Autodesk Fusion 360 part; units mm, degrees
note: some values were not read from the file. Chosen so that the rebuilt part matches the saved one: which pieces of a blend or face edit are solid.
(part 3 of 4)
  arc A691 (-206.3206, 126.4632) -> (-207.0079, 125.7759) centre (-206.5811, 126.0364) ccw
  arc A692 (-206.3206, 126.4632) -> (-206.1643, 126.4193) centre (-206.1643, 126.7193) ccw
  line L408 (-206.1643, 126.4193) -> (-205.2639, 126.4193)
  line L409 (-205.2639, 126.4193) -> (-204.3636, 126.4193)
  arc A693 (-204.3636, 126.4193) -> (-204.2073, 126.4632) centre (-204.3636, 126.7193) ccw
  arc A694 (-203.52, 125.7759) -> (-204.2073, 126.4632) centre (-203.9468, 126.0364) ccw
  arc A695 (-203.52, 125.7759) -> (-203.5639, 125.6196) centre (-203.2639, 125.6196) ccw
  line L410 (-203.5639, 125.6196) -> (-203.5639, 124.9193)
  line L411 (-203.5639, 124.9193) -> (-203.5639, 124.2189)
  arc A696 (-203.5639, 124.2189) -> (-203.52, 124.0626) centre (-203.2639, 124.2189) ccw
  arc A697 (-223.2573, 123.3754) -> (-222.57, 124.0626) centre (-222.9968, 123.8021) ccw
  arc A698 (-223.2573, 123.3754) -> (-223.4136, 123.4193) centre (-223.4135, 123.1196) ccw
  line L412 (-223.4136, 123.4193) -> (-224.3139, 123.4193)
  line L413 (-224.3139, 123.4193) -> (-225.2143, 123.4193)
  arc A699 (-225.2143, 123.4193) -> (-225.3706, 123.3754) centre (-225.2143, 123.1193) ccw
  arc A700 (-226.0579, 124.0626) -> (-225.3706, 123.3754) centre (-225.6311, 123.8021) ccw
  arc A701 (-226.0579, 124.0626) -> (-226.0139, 124.2189) centre (-226.3139, 124.2189) ccw
  line L414 (-226.0139, 124.2189) -> (-226.0139, 124.9193)
  line L415 (-226.0139, 124.9193) -> (-226.0139, 125.6196)
  arc A702 (-226.0139, 125.6196) -> (-226.0579, 125.7759) centre (-226.3139, 125.6196) ccw
  arc A703 (-225.3706, 126.4632) -> (-226.0579, 125.7759) centre (-225.6311, 126.0364) ccw
  arc A704 (-225.3706, 126.4632) -> (-225.2143, 126.4193) centre (-225.2143, 126.7193) ccw
  line L416 (-225.2143, 126.4193) -> (-224.3139, 126.4193)
  line L417 (-224.3139, 126.4193) -> (-223.4136, 126.4193)
  arc A705 (-223.4136, 126.4193) -> (-223.2573, 126.4632) centre (-223.4136, 126.7193) ccw
  arc A706 (-222.57, 125.7759) -> (-223.2573, 126.4632) centre (-222.9968, 126.0364) ccw
  arc A707 (-222.57, 125.7759) -> (-222.6139, 125.6196) centre (-222.3139, 125.6196) ccw
  line L418 (-222.6139, 125.6196) -> (-222.6139, 124.9193)
  line L419 (-222.6139, 124.9193) -> (-222.6139, 124.2189)
  arc A708 (-222.6139, 124.2189) -> (-222.57, 124.0626) centre (-222.3139, 124.2189) ccw
  circle A709 centre (-191.2939, 119.8393) radius 0.875
  circle A710 centre (-200.1839, 119.8393) radius 0.875
  circle A711 centre (-205.2639, 119.8393) radius 1.9939
  circle A712 centre (-201.4539, 117.2993) radius 1.5
  circle A713 centre (-188.7539, 114.7593) radius 1.5
  circle A714 centre (-210.3439, 119.8393) radius 0.875
  circle A715 centre (-219.2339, 119.8393) radius 0.875
  circle A716 centre (-224.3139, 119.8393) radius 1.9939
  circle A717 centre (-220.5039, 117.2993) radius 1.5
  circle A718 centre (-207.8039, 114.7593) radius 1.5
  arc A719 (-156.5823, 104.3254) -> (-155.895, 105.0126) centre (-156.3218, 104.7521) ccw
  arc A720 (-156.5823, 104.3254) -> (-156.7386, 104.3693) centre (-156.7385, 104.0696) ccw
  line L420 (-156.7386, 104.3693) -> (-157.6389, 104.3693)
  line L421 (-157.6389, 104.3693) -> (-158.5393, 104.3693)
  arc A721 (-158.5393, 104.3693) -> (-158.6956, 104.3254) centre (-158.5393, 104.0693) ccw
  arc A722 (-159.3829, 105.0126) -> (-158.6956, 104.3254) centre (-158.9561, 104.7521) ccw
  arc A723 (-159.3829, 105.0126) -> (-159.3389, 105.1689) centre (-159.6389, 105.1689) ccw
  line L422 (-159.3389, 105.1689) -> (-159.3389, 105.8693)
  line L423 (-159.3389, 105.8693) -> (-159.3389, 106.5696)
  arc A724 (-159.3389, 106.5696) -> (-159.3829, 106.7259) centre (-159.6389, 106.5696) ccw
  arc A725 (-158.6956, 107.4132) -> (-159.3829, 106.7259) centre (-158.9561, 106.9864) ccw
  arc A726 (-158.6956, 107.4132) -> (-158.5393, 107.3693) centre (-158.5393, 107.6693) ccw
  line L424 (-158.5393, 107.3693) -> (-157.6389, 107.3693)
  line L425 (-157.6389, 107.3693) -> (-156.7386, 107.3693)
  arc A727 (-156.7386, 107.3693) -> (-156.5823, 107.4132) centre (-156.7386, 107.6693) ccw
  arc A728 (-155.895, 106.7259) -> (-156.5823, 107.4132) centre (-156.3218, 106.9864) ccw
  arc A729 (-155.895, 106.7259) -> (-155.9389, 106.5696) centre (-155.6389, 106.5696) ccw
  line L426 (-155.9389, 106.5696) -> (-155.9389, 105.8693)
  line L427 (-155.9389, 105.8693) -> (-155.9389, 105.1689)
  arc A730 (-155.9389, 105.1689) -> (-155.895, 105.0126) centre (-155.6389, 105.1689) ccw
  arc A731 (-175.6323, 104.3254) -> (-174.945, 105.0126) centre (-175.3718, 104.7521) ccw
  arc A732 (-175.6323, 104.3254) -> (-175.7886, 104.3693) centre (-175.7885, 104.0696) ccw
  line L428 (-175.7886, 104.3693) -> (-176.6889, 104.3693)
  line L429 (-176.6889, 104.3693) -> (-177.5893, 104.3693)
  arc A733 (-177.5893, 104.3693) -> (-177.7456, 104.3254) centre (-177.5893, 104.0693) ccw
  arc A734 (-178.4329, 105.0126) -> (-177.7456, 104.3254) centre (-178.0061, 104.7521) ccw
  arc A735 (-178.4329, 105.0126) -> (-178.3889, 105.1689) centre (-178.6889, 105.1689) ccw
  line L430 (-178.3889, 105.1689) -> (-178.3889, 105.8693)
  line L431 (-178.3889, 105.8693) -> (-178.3889, 106.5696)
  arc A736 (-178.3889, 106.5696) -> (-178.4329, 106.7259) centre (-178.6889, 106.5696) ccw
  arc A737 (-177.7456, 107.4132) -> (-178.4329, 106.7259) centre (-178.0061, 106.9864) ccw
  arc A738 (-177.7456, 107.4132) -> (-177.5893, 107.3693) centre (-177.5893, 107.6693) ccw
  line L432 (-177.5893, 107.3693) -> (-176.6889, 107.3693)
  line L433 (-176.6889, 107.3693) -> (-175.7886, 107.3693)
  arc A739 (-175.7886, 107.3693) -> (-175.6323, 107.4132) centre (-175.7886, 107.6693) ccw
  arc A740 (-174.945, 106.7259) -> (-175.6323, 107.4132) centre (-175.3718, 106.9864) ccw
  arc A741 (-174.945, 106.7259) -> (-174.9889, 106.5696) centre (-174.6889, 106.5696) ccw
  line L434 (-174.9889, 106.5696) -> (-174.9889, 105.8693)
  line L435 (-174.9889, 105.8693) -> (-174.9889, 105.1689)
  arc A742 (-174.9889, 105.1689) -> (-174.945, 105.0126) centre (-174.6889, 105.1689) ccw
  circle A743 centre (-152.5589, 100.7893) radius 0.875
  circle A744 centre (-153.8289, 98.2493) radius 1.5
  circle A745 centre (-157.6389, 100.7893) radius 1.9939
  circle A746 centre (-162.7189, 100.7893) radius 0.875
  circle A747 centre (-171.6089, 100.7893) radius 0.875
  circle A748 centre (-172.8789, 98.2493) radius 1.5
  circle A749 centre (-176.6889, 100.7893) radius 1.9939
  circle A750 centre (-181.7689, 100.7893) radius 0.875
  arc A751 (-194.6823, 104.3254) -> (-193.995, 105.0126) centre (-194.4218, 104.7521) ccw
  arc A752 (-194.6823, 104.3254) -> (-194.8386, 104.3693) centre (-194.8385, 104.0696) ccw
  line L436 (-194.8386, 104.3693) -> (-195.7389, 104.3693)
  line L437 (-195.7389, 104.3693) -> (-196.6393, 104.3693)
  arc A753 (-196.6393, 104.3693) -> (-196.7956, 104.3254) centre (-196.6393, 104.0693) ccw
  arc A754 (-197.4829, 105.0126) -> (-196.7956, 104.3254) centre (-197.0561, 104.7521) ccw
  arc A755 (-197.4829, 105.0126) -> (-197.4389, 105.1689) centre (-197.7389, 105.1689) ccw
  line L438 (-197.4389, 105.1689) -> (-197.4389, 105.8693)
  line L439 (-197.4389, 105.8693) -> (-197.4389, 106.5696)
  arc A756 (-197.4389, 106.5696) -> (-197.4829, 106.7259) centre (-197.7389, 106.5696) ccw
  arc A757 (-196.7956, 107.4132) -> (-197.4829, 106.7259) centre (-197.0561, 106.9864) ccw
  arc A758 (-196.7956, 107.4132) -> (-196.6393, 107.3693) centre (-196.6393, 107.6693) ccw
  line L440 (-196.6393, 107.3693) -> (-195.7389, 107.3693)
  line L441 (-195.7389, 107.3693) -> (-194.8386, 107.3693)
  arc A759 (-194.8386, 107.3693) -> (-194.6823, 107.4132) centre (-194.8386, 107.6693) ccw
  arc A760 (-193.995, 106.7259) -> (-194.6823, 107.4132) centre (-194.4218, 106.9864) ccw
  arc A761 (-193.995, 106.7259) -> (-194.0389, 106.5696) centre (-193.7389, 106.5696) ccw
  line L442 (-194.0389, 106.5696) -> (-194.0389, 105.8693)
  line L443 (-194.0389, 105.8693) -> (-194.0389, 105.1689)
  arc A762 (-194.0389, 105.1689) -> (-193.995, 105.0126) centre (-193.7389, 105.1689) ccw
  arc A763 (-213.7323, 104.3254) -> (-213.045, 105.0126) centre (-213.4718, 104.7521) ccw
  arc A764 (-213.7323, 104.3254) -> (-213.8886, 104.3693) centre (-213.8885, 104.0696) ccw
  line L444 (-213.8886, 104.3693) -> (-214.7889, 104.3693)
  line L445 (-214.7889, 104.3693) -> (-215.6893, 104.3693)
  arc A765 (-215.6893, 104.3693) -> (-215.8456, 104.3254) centre (-215.6893, 104.0693) ccw
  arc A766 (-216.5329, 105.0126) -> (-215.8456, 104.3254) centre (-216.1061, 104.7521) ccw
  arc A767 (-216.5329, 105.0126) -> (-216.4889, 105.1689) centre (-216.7889, 105.1689) ccw
  line L446 (-216.4889, 105.1689) -> (-216.4889, 105.8693)
  line L447 (-216.4889, 105.8693) -> (-216.4889, 106.5696)
  arc A768 (-216.4889, 106.5696) -> (-216.5329, 106.7259) centre (-216.7889, 106.5696) ccw
  arc A769 (-215.8456, 107.4132) -> (-216.5329, 106.7259) centre (-216.1061, 106.9864) ccw
  arc A770 (-215.8456, 107.4132) -> (-215.6893, 107.3693) centre (-215.6893, 107.6693) ccw
  line L448 (-215.6893, 107.3693) -> (-214.7889, 107.3693)
  line L449 (-214.7889, 107.3693) -> (-213.8886, 107.3693)
  arc A771 (-213.8886, 107.3693) -> (-213.7323, 107.4132) centre (-213.8886, 107.6693) ccw
  arc A772 (-213.045, 106.7259) -> (-213.7323, 107.4132) centre (-213.4718, 106.9864) ccw
  arc A773 (-213.045, 106.7259) -> (-213.0889, 106.5696) centre (-212.7889, 106.5696) ccw
  line L450 (-213.0889, 106.5696) -> (-213.0889, 105.8693)
  line L451 (-213.0889, 105.8693) -> (-213.0889, 105.1689)
  arc A774 (-213.0889, 105.1689) -> (-213.045, 105.0126) centre (-212.7889, 105.1689) ccw
  circle A775 centre (-190.6589, 100.7893) radius 0.875
  circle A776 centre (-195.7389, 100.7893) radius 1.9939
  circle A777 centre (-191.9289, 98.2493) radius 1.5
  circle A778 centre (-200.8189, 100.7893) radius 0.875
  circle A779 centre (-209.7089, 100.7893) radius 0.875
  circle A780 centre (-214.7889, 100.7893) radius 1.9939
  circle A781 centre (-210.9789, 98.2493) radius 1.5
  circle A782 centre (-219.8689, 100.7893) radius 0.875
  arc A783 (-242.3073, 123.3754) -> (-241.62, 124.0626) centre (-242.0468, 123.8021) ccw
  arc A784 (-242.3073, 123.3754) -> (-242.4636, 123.4193) centre (-242.4635, 123.1196) ccw
  line L452 (-242.4636, 123.4193) -> (-243.3639, 123.4193)
  line L453 (-243.3639, 123.4193) -> (-244.2643, 123.4193)
  arc A785 (-244.2643, 123.4193) -> (-244.4206, 123.3754) centre (-244.2643, 123.1193) ccw
  arc A786 (-245.1079, 124.0626) -> (-244.4206, 123.3754) centre (-244.6811, 123.8021) ccw
  arc A787 (-245.1079, 124.0626) -> (-245.0639, 124.2189) centre (-245.3639, 124.2189) ccw
  line L454 (-245.0639, 124.2189) -> (-245.0639, 124.9193)
  line L455 (-245.0639, 124.9193) -> (-245.0639, 125.6196)
  arc A788 (-245.0639, 125.6196) -> (-245.1079, 125.7759) centre (-245.3639, 125.6196) ccw
  arc A789 (-244.4206, 126.4632) -> (-245.1079, 125.7759) centre (-244.6811, 126.0364) ccw
  arc A790 (-244.4206, 126.4632) -> (-244.2643, 126.4193) centre (-244.2643, 126.7193) ccw
  line L456 (-244.2643, 126.4193) -> (-243.3639, 126.4193)
  line L457 (-243.3639, 126.4193) -> (-242.4636, 126.4193)
  arc A791 (-242.4636, 126.4193) -> (-242.3073, 126.4632) centre (-242.4636, 126.7193) ccw
  arc A792 (-241.62, 125.7759) -> (-242.3073, 126.4632) centre (-242.0468, 126.0364) ccw
  arc A793 (-241.62, 125.7759) -> (-241.6639, 125.6196) centre (-241.3639, 125.6196) ccw
  line L458 (-241.6639, 125.6196) -> (-241.6639, 124.9193)
  line L459 (-241.6639, 124.9193) -> (-241.6639, 124.2189)
  arc A794 (-241.6639, 124.2189) -> (-241.62, 124.0626) centre (-241.3639, 124.2189) ccw
  arc A795 (-261.3573, 123.3754) -> (-260.67, 124.0626) centre (-261.0968, 123.8021) ccw
  arc A796 (-261.3573, 123.3754) -> (-261.5136, 123.4193) centre (-261.5135, 123.1196) ccw
  line L460 (-261.5136, 123.4193) -> (-262.4139, 123.4193)
  line L461 (-262.4139, 123.4193) -> (-263.3143, 123.4193)
  arc A797 (-263.3143, 123.4193) -> (-263.4706, 123.3754) centre (-263.3143, 123.1193) ccw
  arc A798 (-264.1579, 124.0626) -> (-263.4706, 123.3754) centre (-263.7311, 123.8021) ccw
  arc A799 (-264.1579, 124.0626) -> (-264.1139, 124.2189) centre (-264.4139, 124.2189) ccw
  line L462 (-264.1139, 124.2189) -> (-264.1139, 124.9193)
  line L463 (-264.1139, 124.9193) -> (-264.1139, 125.6196)
  arc A800 (-264.1139, 125.6196) -> (-264.1579, 125.7759) centre (-264.4139, 125.6196) ccw
  arc A801 (-263.4706, 126.4632) -> (-264.1579, 125.7759) centre (-263.7311, 126.0364) ccw
  arc A802 (-263.4706, 126.4632) -> (-263.3143, 126.4193) centre (-263.3143, 126.7193) ccw
  line L464 (-263.3143, 126.4193) -> (-262.4139, 126.4193)
  line L465 (-262.4139, 126.4193) -> (-261.5136, 126.4193)
  arc A803 (-261.5136, 126.4193) -> (-261.3573, 126.4632) centre (-261.5136, 126.7193) ccw
  arc A804 (-260.67, 125.7759) -> (-261.3573, 126.4632) centre (-261.0968, 126.0364) ccw
  arc A805 (-260.67, 125.7759) -> (-260.7139, 125.6196) centre (-260.4139, 125.6196) ccw
  line L466 (-260.7139, 125.6196) -> (-260.7139, 124.9193)
  line L467 (-260.7139, 124.9193) -> (-260.7139, 124.2189)
  arc A806 (-260.7139, 124.2189) -> (-260.67, 124.0626) centre (-260.4139, 124.2189) ccw
  circle A807 centre (-229.3939, 119.8393) radius 0.875
  circle A808 centre (-238.2839, 119.8393) radius 0.875
  circle A809 centre (-243.3639, 119.8393) radius 1.9939
  circle A810 centre (-239.5539, 117.2993) radius 1.5
  circle A811 centre (-226.8539, 114.7593) radius 1.5
  circle A812 centre (-245.9039, 114.7593) radius 1.5
  circle A813 centre (-248.4439, 119.8393) radius 0.875
  circle A814 centre (-257.3339, 119.8393) radius 0.875
  circle A815 centre (-262.4139, 119.8393) radius 1.9939
  circle A816 centre (-258.6039, 117.2993) radius 1.5
  circle A817 centre (-264.9539, 114.7593) radius 1.5
  arc A818 (-283.2079, 124.0626) -> (-282.5206, 123.3754) centre (-282.7811, 123.8021) ccw
  arc A819 (-283.2079, 124.0626) -> (-283.1639, 124.2189) centre (-283.4639, 124.2189) ccw
  line L468 (-283.1639, 124.2189) -> (-283.1639, 124.9193)
  line L469 (-283.1639, 124.9193) -> (-283.1639, 125.6196)
  arc A820 (-283.1639, 125.6196) -> (-283.2079, 125.7759) centre (-283.4639, 125.6196) ccw
  arc A821 (-282.5206, 126.4632) -> (-283.2079, 125.7759) centre (-282.7811, 126.0364) ccw
  arc A822 (-282.5206, 126.4632) -> (-282.3643, 126.4193) centre (-282.3643, 126.7193) ccw
  line L470 (-282.3643, 126.4193) -> (-281.4639, 126.4193)
  line L471 (-281.4639, 126.4193) -> (-280.5636, 126.4193)
  arc A823 (-280.5636, 126.4193) -> (-280.4073, 126.4632) centre (-280.5636, 126.7193) ccw
  arc A824 (-279.72, 125.7759) -> (-280.4073, 126.4632) centre (-280.1468, 126.0364) ccw
  arc A825 (-279.72, 125.7759) -> (-279.7639, 125.6196) centre (-279.4639, 125.6196) ccw
  line L472 (-279.7639, 125.6196) -> (-279.7639, 124.9193)
  line L473 (-279.7639, 124.9193) -> (-279.7639, 124.2189)
  arc A826 (-279.7639, 124.2189) -> (-279.72, 124.0626) centre (-279.4639, 124.2189) ccw
  arc A827 (-280.4073, 123.3754) -> (-279.72, 124.0626) centre (-280.1468, 123.8021) ccw
  arc A828 (-280.4073, 123.3754) -> (-280.5636, 123.4193) centre (-280.5635, 123.1196) ccw
  line L474 (-280.5636, 123.4193) -> (-281.4639, 123.4193)
  line L475 (-281.4639, 123.4193) -> (-282.3643, 123.4193)
  arc A829 (-282.3643, 123.4193) -> (-282.5206, 123.3754) centre (-282.3643, 123.1193) ccw
  arc A830 (-302.2579, 124.0626) -> (-301.5706, 123.3754) centre (-301.8311, 123.8021) ccw
  arc A831 (-302.2579, 124.0626) -> (-302.2139, 124.2189) centre (-302.5139, 124.2189) ccw
  line L476 (-302.2139, 124.2189) -> (-302.2139, 124.9193)
  line L477 (-302.2139, 124.9193) -> (-302.2139, 125.6196)
  arc A832 (-302.2139, 125.6196) -> (-302.2579, 125.7759) centre (-302.5139, 125.6196) ccw
  arc A833 (-301.5706, 126.4632) -> (-302.2579, 125.7759) centre (-301.8311, 126.0364) ccw
  arc A834 (-301.5706, 126.4632) -> (-301.4143, 126.4193) centre (-301.4143, 126.7193) ccw
  line L478 (-301.4143, 126.4193) -> (-300.5139, 126.4193)
  line L479 (-300.5139, 126.4193) -> (-299.6136, 126.4193)
  arc A835 (-299.6136, 126.4193) -> (-299.4573, 126.4632) centre (-299.6136, 126.7193) ccw
  arc A836 (-298.77, 125.7759) -> (-299.4573, 126.4632) centre (-299.1968, 126.0364) ccw
  arc A837 (-298.77, 125.7759) -> (-298.8139, 125.6196) centre (-298.5139, 125.6196) ccw
  line L480 (-298.8139, 125.6196) -> (-298.8139, 124.9193)
  line L481 (-298.8139, 124.9193) -> (-298.8139, 124.2189)
  arc A838 (-298.8139, 124.2189) -> (-298.77, 124.0626) centre (-298.5139, 124.2189) ccw
  arc A839 (-299.4573, 123.3754) -> (-298.77, 124.0626) centre (-299.1968, 123.8021) ccw
  arc A840 (-299.4573, 123.3754) -> (-299.6136, 123.4193) centre (-299.6135, 123.1196) ccw
  line L482 (-299.6136, 123.4193) -> (-300.5139, 123.4193)
  line L483 (-300.5139, 123.4193) -> (-301.4143, 123.4193)
  arc A841 (-301.4143, 123.4193) -> (-301.5706, 123.3754) centre (-301.4143, 123.1193) ccw
  circle A842 centre (-267.4939, 119.8393) radius 0.875
  circle A843 centre (-276.3839, 119.8393) radius 0.875
  circle A844 centre (-281.4639, 119.8393) radius 1.9939
  circle A845 centre (-277.6539, 117.2993) radius 1.5
  circle A846 centre (-284.0039, 114.7593) radius 1.5
  circle A847 centre (-286.5439, 119.8393) radius 0.875
  circle A848 centre (-295.4339, 119.8393) radius 0.875
  circle A849 centre (-300.5139, 119.8393) radius 1.9939
  circle A850 centre (-296.7039, 117.2993) radius 1.5
  circle A851 centre (-303.0539, 114.7593) radius 1.5
  arc A852 (-232.7823, 104.3254) -> (-232.095, 105.0126) centre (-232.5218, 104.7521) ccw
  arc A853 (-232.7823, 104.3254) -> (-232.9386, 104.3693) centre (-232.9385, 104.0696) ccw
  line L484 (-232.9386, 104.3693) -> (-233.8389, 104.3693)
  line L485 (-233.8389, 104.3693) -> (-234.7393, 104.3693)
  arc A854 (-234.7393, 104.3693) -> (-234.8956, 104.3254) centre (-234.7393, 104.0693) ccw
  arc A855 (-235.5829, 105.0126) -> (-234.8956, 104.3254) centre (-235.1561, 104.7521) ccw
  arc A856 (-235.5829, 105.0126) -> (-235.5389, 105.1689) centre (-235.8389, 105.1689) ccw
  line L486 (-235.5389, 105.1689) -> (-235.5389, 105.8693)
  line L487 (-235.5389, 105.8693) -> (-235.5389, 106.5696)
  arc A857 (-235.5389, 106.5696) -> (-235.5829, 106.7259) centre (-235.8389, 106.5696) ccw
  arc A858 (-234.8956, 107.4132) -> (-235.5829, 106.7259) centre (-235.1561, 106.9864) ccw
  arc A859 (-234.8956, 107.4132) -> (-234.7393, 107.3693) centre (-234.7393, 107.6693) ccw
  line L488 (-234.7393, 107.3693) -> (-233.8389, 107.3693)
  line L489 (-233.8389, 107.3693) -> (-232.9386, 107.3693)
  arc A860 (-232.9386, 107.3693) -> (-232.7823, 107.4132) centre (-232.9386, 107.6693) ccw
  arc A861 (-232.095, 106.7259) -> (-232.7823, 107.4132) centre (-232.5218, 106.9864) ccw
  arc A862 (-232.095, 106.7259) -> (-232.1389, 106.5696) centre (-231.8389, 106.5696) ccw
  line L490 (-232.1389, 106.5696) -> (-232.1389, 105.8693)
  line L491 (-232.1389, 105.8693) -> (-232.1389, 105.1689)
  arc A863 (-232.1389, 105.1689) -> (-232.095, 105.0126) centre (-231.8389, 105.1689) ccw
  arc A864 (-251.8323, 104.3254) -> (-251.145, 105.0126) centre (-251.5718, 104.7521) ccw
  arc A865 (-251.8323, 104.3254) -> (-251.9886, 104.3693) centre (-251.9885, 104.0696) ccw
  line L492 (-251.9886, 104.3693) -> (-252.8889, 104.3693)
  line L493 (-252.8889, 104.3693) -> (-253.7893, 104.3693)
  arc A866 (-253.7893, 104.3693) -> (-253.9456, 104.3254) centre (-253.7893, 104.0693) ccw
  arc A867 (-254.6329, 105.0126) -> (-253.9456, 104.3254) centre (-254.2061, 104.7521) ccw
  arc A868 (-254.6329, 105.0126) -> (-254.5889, 105.1689) centre (-254.8889, 105.1689) ccw
  line L494 (-254.5889, 105.1689) -> (-254.5889, 105.8693)
  line L495 (-254.5889, 105.8693) -> (-254.5889, 106.5696)
  arc A869 (-254.5889, 106.5696) -> (-254.6329, 106.7259) centre (-254.8889, 106.5696) ccw
  arc A870 (-253.9456, 107.4132) -> (-254.6329, 106.7259) centre (-254.2061, 106.9864) ccw
  arc A871 (-253.9456, 107.4132) -> (-253.7893, 107.3693) centre (-253.7893, 107.6693) ccw
  line L496 (-253.7893, 107.3693) -> (-252.8889, 107.3693)
  line L497 (-252.8889, 107.3693) -> (-251.9886, 107.3693)
  arc A872 (-251.9886, 107.3693) -> (-251.8323, 107.4132) centre (-251.9886, 107.6693) ccw
  arc A873 (-251.145, 106.7259) -> (-251.8323, 107.4132) centre (-251.5718, 106.9864) ccw
  arc A874 (-251.145, 106.7259) -> (-251.1889, 106.5696) centre (-250.8889, 106.5696) ccw
  line L498 (-251.1889, 106.5696) -> (-251.1889, 105.8693)
  line L499 (-251.1889, 105.8693) -> (-251.1889, 105.1689)
  arc A875 (-251.1889, 105.1689) -> (-251.145, 105.0126) centre (-250.8889, 105.1689) ccw
  circle A876 centre (-228.7589, 100.7893) radius 0.875
  circle A877 centre (-233.8389, 100.7893) radius 1.9939
  circle A878 centre (-230.0289, 98.2493) radius 1.5
  circle A879 centre (-238.9189, 100.7893) radius 0.875
  circle A880 centre (-247.8089, 100.7893) radius 0.875
  circle A881 centre (-252.8889, 100.7893) radius 1.9939
  circle A882 centre (-249.0789, 98.2493) radius 1.5
  circle A883 centre (-257.9689, 100.7893) radius 0.875
  arc A884 (-270.8823, 104.3254) -> (-270.195, 105.0126) centre (-270.6218, 104.7521) ccw
  arc A885 (-270.8823, 104.3254) -> (-271.0386, 104.3693) centre (-271.0385, 104.0696) ccw
  line L500 (-271.0386, 104.3693) -> (-271.9389, 104.3693)
  line L501 (-271.9389, 104.3693) -> (-272.8393, 104.3693)
  arc A886 (-272.8393, 104.3693) -> (-272.9956, 104.3254) centre (-272.8393, 104.0693) ccw
  arc A887 (-273.6829, 105.0126) -> (-272.9956, 104.3254) centre (-273.2561, 104.7521) ccw
  arc A888 (-273.6829, 105.0126) -> (-273.6389, 105.1689) centre (-273.9389, 105.1689) ccw
  line L502 (-273.6389, 105.1689) -> (-273.6389, 105.8693)
  line L503 (-273.6389, 105.8693) -> (-273.6389, 106.5696)
  arc A889 (-273.6389, 106.5696) -> (-273.6829, 106.7259) centre (-273.9389, 106.5696) ccw
  arc A890 (-272.9956, 107.4132) -> (-273.6829, 106.7259) centre (-273.2561, 106.9864) ccw
  arc A891 (-272.9956, 107.4132) -> (-272.8393, 107.3693) centre (-272.8393, 107.6693) ccw
  line L504 (-272.8393, 107.3693) -> (-271.9389, 107.3693)
  line L505 (-271.9389, 107.3693) -> (-271.0386, 107.3693)
  arc A892 (-271.0386, 107.3693) -> (-270.8823, 107.4132) centre (-271.0386, 107.6693) ccw
  arc A893 (-270.195, 106.7259) -> (-270.8823, 107.4132) centre (-270.6218, 106.9864) ccw
  arc A894 (-270.195, 106.7259) -> (-270.2389, 106.5696) centre (-269.9389, 106.5696) ccw
  line L506 (-270.2389, 106.5696) -> (-270.2389, 105.8693)
  line L507 (-270.2389, 105.8693) -> (-270.2389, 105.1689)
  arc A895 (-270.2389, 105.1689) -> (-270.195, 105.0126) centre (-269.9389, 105.1689) ccw
  arc A896 (-292.7329, 105.0126) -> (-292.0456, 104.3254) centre (-292.3061, 104.7521) ccw
  arc A897 (-292.7329, 105.0126) -> (-292.6889, 105.1689) centre (-292.9889, 105.1689) ccw
  line L508 (-292.6889, 105.1689) -> (-292.6889, 105.8693)
  line L509 (-292.6889, 105.8693) -> (-292.6889, 106.5696)
  arc A898 (-292.6889, 106.5696) -> (-292.7329, 106.7259) centre (-292.9889, 106.5696) ccw
  arc A899 (-292.0456, 107.4132) -> (-292.7329, 106.7259) centre (-292.3061, 106.9864) ccw
  arc A900 (-292.0456, 107.4132) -> (-291.8893, 107.3693) centre (-291.8893, 107.6693) ccw
  line L510 (-291.8893, 107.3693) -> (-290.9889, 107.3693)
  line L511 (-290.9889, 107.3693) -> (-290.0886, 107.3693)
  arc A901 (-290.0886, 107.3693) -> (-289.9323, 107.4132) centre (-290.0886, 107.6693) ccw
  arc A902 (-289.245, 106.7259) -> (-289.9323, 107.4132) centre (-289.6718, 106.9864) ccw
  arc A903 (-289.245, 106.7259) -> (-289.2889, 106.5696) centre (-288.9889, 106.5696) ccw
  line L512 (-289.2889, 106.5696) -> (-289.2889, 105.8693)
  line L513 (-289.2889, 105.8693) -> (-289.2889, 105.1689)
  arc A904 (-289.2889, 105.1689) -> (-289.245, 105.0126) centre (-288.9889, 105.1689) ccw
  arc A905 (-289.9323, 104.3254) -> (-289.245, 105.0126) centre (-289.6718, 104.7521) ccw
  arc A906 (-289.9323, 104.3254) -> (-290.0886, 104.3693) centre (-290.0885, 104.0696) ccw
  line L514 (-290.0886, 104.3693) -> (-290.9889, 104.3693)
  line L515 (-290.9889, 104.3693) -> (-291.8893, 104.3693)
  arc A907 (-291.8893, 104.3693) -> (-292.0456, 104.3254) centre (-291.8893, 104.0693) ccw
  circle A908 centre (-266.8589, 100.7893) radius 0.875
  circle A909 centre (-271.9389, 100.7893) radius 1.9939
  circle A910 centre (-268.1289, 98.2493) radius 1.5
  circle A911 centre (-277.0189, 100.7893) radius 0.875
  circle A912 centre (-285.9089, 100.7893) radius 0.875
  circle A913 centre (-290.9889, 100.7893) radius 1.9939
  circle A914 centre (-287.1789, 98.2493) radius 1.5
  circle A915 centre (-296.0689, 100.7893) radius 0.875
  circle A916 centre (-304.9589, 100.7893) radius 0.875
  circle A917 centre (-160.1789, 95.7093) radius 1.5
  circle A918 centre (-179.2289, 95.7093) radius 1.5
  arc A919 (-156.5823, 80.5129) -> (-155.895, 81.2001) centre (-156.3218, 80.9396) ccw
  arc A920 (-156.5823, 80.5129) -> (-156.7386, 80.5568) centre (-156.7385, 80.2571) ccw
  line L516 (-156.7386, 80.5568) -> (-157.6389, 80.5568)
  line L517 (-157.6389, 80.5568) -> (-158.5393, 80.5568)
  arc A921 (-158.5393, 80.5568) -> (-158.6956, 80.5129) centre (-158.5393, 80.2568) ccw
  arc A922 (-159.3829, 81.2001) -> (-158.6956, 80.5129) centre (-158.9561, 80.9396) ccw
  arc A923 (-159.3829, 81.2001) -> (-159.3389, 81.3564) centre (-159.6389, 81.3564) ccw
  line L518 (-159.3389, 81.3564) -> (-159.3389, 82.0568)
  line L519 (-159.3389, 82.0568) -> (-159.3389, 82.7571)
  arc A924 (-159.3389, 82.7571) -> (-159.3829, 82.9134) centre (-159.6389, 82.7571) ccw
  arc A925 (-158.6956, 83.6007) -> (-159.3829, 82.9134) centre (-158.9561, 83.1739) ccw
  arc A926 (-158.6956, 83.6007) -> (-158.5393, 83.5568) centre (-158.5393, 83.8568) ccw
  line L520 (-158.5393, 83.5568) -> (-157.6389, 83.5568)
  line L521 (-157.6389, 83.5568) -> (-156.7386, 83.5568)
  arc A927 (-156.7386, 83.5568) -> (-156.5823, 83.6007) centre (-156.7386, 83.8568) ccw
  arc A928 (-155.895, 82.9134) -> (-156.5823, 83.6007) centre (-156.3218, 83.1739) ccw
  arc A929 (-155.895, 82.9134) -> (-155.9389, 82.7571) centre (-155.6389, 82.7571) ccw
  line L522 (-155.9389, 82.7571) -> (-155.9389, 82.0568)
  line L523 (-155.9389, 82.0568) -> (-155.9389, 81.3564)
  arc A930 (-155.9389, 81.3564) -> (-155.895, 81.2001) centre (-155.6389, 81.3564) ccw
  circle A931 centre (-169.5452, 88.883) radius 1.1
  arc A932 (-180.3948, 80.5129) -> (-179.7075, 81.2001) centre (-180.1343, 80.9396) ccw
  arc A933 (-180.3948, 80.5129) -> (-180.5511, 80.5568) centre (-180.551, 80.2571) ccw
  line L524 (-180.5511, 80.5568) -> (-181.4514, 80.5568)
  line L525 (-181.4514, 80.5568) -> (-182.3518, 80.5568)
  arc A934 (-182.3518, 80.5568) -> (-182.5081, 80.5129) centre (-182.3518, 80.2568) ccw
  arc A935 (-183.1954, 81.2001) -> (-182.5081, 80.5129) centre (-182.7686, 80.9396) ccw
  arc A936 (-183.1954, 81.2001) -> (-183.1514, 81.3564) centre (-183.4514, 81.3564) ccw
  line L526 (-183.1514, 81.3564) -> (-183.1514, 82.0568)
  line L527 (-183.1514, 82.0568) -> (-183.1514, 82.7571)
  arc A937 (-183.1514, 82.7571) -> (-183.1954, 82.9134) centre (-183.4514, 82.7571) ccw
  arc A938 (-182.5081, 83.6007) -> (-183.1954, 82.9134) centre (-182.7686, 83.1739) ccw
  arc A939 (-182.5081, 83.6007) -> (-182.3518, 83.5568) centre (-182.3518, 83.8568) ccw
  line L528 (-182.3518, 83.5568) -> (-181.4514, 83.5568)
  line L529 (-181.4514, 83.5568) -> (-180.5511, 83.5568)
  arc A940 (-180.5511, 83.5568) -> (-180.3948, 83.6007) centre (-180.5511, 83.8568) ccw
  arc A941 (-179.7075, 82.9134) -> (-180.3948, 83.6007) centre (-180.1343, 83.1739) ccw
  arc A942 (-179.7075, 82.9134) -> (-179.7514, 82.7571) centre (-179.4514, 82.7571) ccw
  line L530 (-179.7514, 82.7571) -> (-179.7514, 82.0568)
  line L531 (-179.7514, 82.0568) -> (-179.7514, 81.3564)
  arc A943 (-179.7514, 81.3564) -> (-179.7075, 81.2001) centre (-179.4514, 81.3564) ccw
  circle A944 centre (-198.2789, 95.7093) radius 1.5
  circle A945 centre (-217.3289, 95.7093) radius 1.5
  arc A946 (-199.4448, 80.5129) -> (-198.7575, 81.2001) centre (-199.1843, 80.9396) ccw
  arc A947 (-199.4448, 80.5129) -> (-199.6011, 80.5568) centre (-199.601, 80.2571) ccw
  line L532 (-199.6011, 80.5568) -> (-200.5014, 80.5568)
  line L533 (-200.5014, 80.5568) -> (-201.4018, 80.5568)
  arc A948 (-201.4018, 80.5568) -> (-201.5581, 80.5129) centre (-201.4018, 80.2568) ccw
  arc A949 (-202.2454, 81.2001) -> (-201.5581, 80.5129) centre (-201.8186, 80.9396) ccw
  arc A950 (-202.2454, 81.2001) -> (-202.2014, 81.3564) centre (-202.5014, 81.3564) ccw
  line L534 (-202.2014, 81.3564) -> (-202.2014, 82.0568)
  line L535 (-202.2014, 82.0568) -> (-202.2014, 82.7571)
  arc A951 (-202.2014, 82.7571) -> (-202.2454, 82.9134) centre (-202.5014, 82.7571) ccw
  arc A952 (-201.5581, 83.6007) -> (-202.2454, 82.9134) centre (-201.8186, 83.1739) ccw
  arc A953 (-201.5581, 83.6007) -> (-201.4018, 83.5568) centre (-201.4018, 83.8568) ccw
  line L536 (-201.4018, 83.5568) -> (-200.5014, 83.5568)
  line L537 (-200.5014, 83.5568) -> (-199.6011, 83.5568)
  arc A954 (-199.6011, 83.5568) -> (-199.4448, 83.6007) centre (-199.6011, 83.8568) ccw
  arc A955 (-198.7575, 82.9134) -> (-199.4448, 83.6007) centre (-199.1843, 83.1739) ccw
  arc A956 (-198.7575, 82.9134) -> (-198.8014, 82.7571) centre (-198.5014, 82.7571) ccw
  line L538 (-198.8014, 82.7571) -> (-198.8014, 82.0568)
  line L539 (-198.8014, 82.0568) -> (-198.8014, 81.3564)
  arc A957 (-198.8014, 81.3564) -> (-198.7575, 81.2001) centre (-198.5014, 81.3564) ccw
  arc A958 (-218.4948, 80.5129) -> (-217.8075, 81.2001) centre (-218.2343, 80.9396) ccw
  arc A959 (-218.4948, 80.5129) -> (-218.6511, 80.5568) centre (-218.651, 80.2571) ccw
  line L540 (-218.6511, 80.5568) -> (-219.5514, 80.5568)
  line L541 (-219.5514, 80.5568) -> (-220.4518, 80.5568)
  arc A960 (-220.4518, 80.5568) -> (-220.6081, 80.5129) centre (-220.4518, 80.2568) ccw
  arc A961 (-221.2954, 81.2001) -> (-220.6081, 80.5129) centre (-220.8686, 80.9396) ccw
  arc A962 (-221.2954, 81.2001) -> (-221.2514, 81.3564) centre (-221.5514, 81.3564) ccw
  line L542 (-221.2514, 81.3564) -> (-221.2514, 82.0568)
  line L543 (-221.2514, 82.0568) -> (-221.2514, 82.7571)
  arc A963 (-221.2514, 82.7571) -> (-221.2954, 82.9134) centre (-221.5514, 82.7571) ccw
  arc A964 (-220.6081, 83.6007) -> (-221.2954, 82.9134) centre (-220.8686, 83.1739) ccw
  arc A965 (-220.6081, 83.6007) -> (-220.4518, 83.5568) centre (-220.4518, 83.8568) ccw
  line L544 (-220.4518, 83.5568) -> (-219.5514, 83.5568)
  line L545 (-219.5514, 83.5568) -> (-218.6511, 83.5568)
  arc A966 (-218.6511, 83.5568) -> (-218.4948, 83.6007) centre (-218.6511, 83.8568) ccw
  arc A967 (-217.8075, 82.9134) -> (-218.4948, 83.6007) centre (-218.2343, 83.1739) ccw
  arc A968 (-217.8075, 82.9134) -> (-217.8514, 82.7571) centre (-217.5514, 82.7571) ccw
  line L546 (-217.8514, 82.7571) -> (-217.8514, 82.0568)
  line L547 (-217.8514, 82.0568) -> (-217.8514, 81.3564)
  arc A969 (-217.8514, 81.3564) -> (-217.8075, 81.2001) centre (-217.5514, 81.3564) ccw
  circle A970 centre (-152.5589, 76.9768) radius 0.875
  circle A971 centre (-153.8289, 74.4368) radius 1.5
  circle A972 centre (-157.6389, 76.9768) radius 1.9939
  circle A973 centre (-162.7189, 76.9768) radius 0.875
  circle A974 centre (-176.3714, 76.9768) radius 0.875
  circle A975 centre (-181.4514, 76.9768) radius 1.9939
  circle A976 centre (-186.5314, 76.9768) radius 0.875
  circle A977 centre (-177.6414, 74.4368) radius 1.5
  circle A978 centre (-160.1789, 71.8968) radius 1.5
  circle A979 centre (-148.1139, 67.4518) radius 1.1
  circle A980 centre (-183.9914, 71.8968) radius 1.5
  circle A981 centre (-169.5452, 67.4518) radius 1.1
  circle A982 centre (-195.4214, 76.9768) radius 0.875
  circle A983 centre (-200.5014, 76.9768) radius 1.9939
  circle A984 centre (-205.5814, 76.9768) radius 0.875
  circle A985 centre (-196.6914, 74.4368) radius 1.5
  circle A986 centre (-214.4714, 76.9768) radius 0.875
  circle A987 centre (-215.7414, 74.4368) radius 1.5
  circle A988 centre (-219.5514, 76.9768) radius 1.9939
  circle A989 centre (-224.6314, 76.9768) radius 0.875
  circle A990 centre (-203.0414, 71.8968) radius 1.5
  circle A991 centre (-222.0914, 71.8968) radius 1.5
  circle A992 centre (-236.3789, 95.7093) radius 1.5
  circle A993 centre (-255.4289, 95.7093) radius 1.5
  arc A994 (-237.5448, 80.5129) -> (-236.8575, 81.2001) centre (-237.2843, 80.9396) ccw
  arc A995 (-237.5448, 80.5129) -> (-237.7011, 80.5568) centre (-237.701, 80.2571) ccw
  line L548 (-237.7011, 80.5568) -> (-238.6014, 80.5568)
  line L549 (-238.6014, 80.5568) -> (-239.5018, 80.5568)
  arc A996 (-239.5018, 80.5568) -> (-239.6581, 80.5129) centre (-239.5018, 80.2568) ccw
  arc A997 (-240.3454, 81.2001) -> (-239.6581, 80.5129) centre (-239.9186, 80.9396) ccw
  arc A998 (-240.3454, 81.2001) -> (-240.3014, 81.3564) centre (-240.6014, 81.3564) ccw
  line L550 (-240.3014, 81.3564) -> (-240.3014, 82.0568)
  line L551 (-240.3014, 82.0568) -> (-240.3014, 82.7571)
  arc A999 (-240.3014, 82.7571) -> (-240.3454, 82.9134) centre (-240.6014, 82.7571) ccw
  arc A1000 (-239.6581, 83.6007) -> (-240.3454, 82.9134) centre (-239.9186, 83.1739) ccw
  arc A1001 (-239.6581, 83.6007) -> (-239.5018, 83.5568) centre (-239.5018, 83.8568) ccw
  line L552 (-239.5018, 83.5568) -> (-238.6014, 83.5568)
  line L553 (-238.6014, 83.5568) -> (-237.7011, 83.5568)
  arc A1002 (-237.7011, 83.5568) -> (-237.5448, 83.6007) centre (-237.7011, 83.8568) ccw
  arc A1003 (-236.8575, 82.9134) -> (-237.5448, 83.6007) centre (-237.2843, 83.1739) ccw
  arc A1004 (-236.8575, 82.9134) -> (-236.9014, 82.7571) centre (-236.6014, 82.7571) ccw
  line L554 (-236.9014, 82.7571) -> (-236.9014, 82.0568)
  line L555 (-236.9014, 82.0568) -> (-236.9014, 81.3564)
  arc A1005 (-236.9014, 81.3564) -> (-236.8575, 81.2001) centre (-236.6014, 81.3564) ccw
  circle A1006 centre (-250.5077, 88.883) radius 1.1
  arc A1007 (-261.3573, 80.5129) -> (-260.67, 81.2001) centre (-261.0968, 80.9396) ccw
  arc A1008 (-261.3573, 80.5129) -> (-261.5136, 80.5568) centre (-261.5135, 80.2571) ccw
  line L556 (-261.5136, 80.5568) -> (-262.4139, 80.5568)
  line L557 (-262.4139, 80.5568) -> (-263.3143, 80.5568)
  arc A1009 (-263.3143, 80.5568) -> (-263.4706, 80.5129) centre (-263.3143, 80.2568) ccw
  arc A1010 (-264.1579, 81.2001) -> (-263.4706, 80.5129) centre (-263.7311, 80.9396) ccw
  arc A1011 (-264.1579, 81.2001) -> (-264.1139, 81.3564) centre (-264.4139, 81.3564) ccw
  line L558 (-264.1139, 81.3564) -> (-264.1139, 82.0568)
  line L559 (-264.1139, 82.0568) -> (-264.1139, 82.7571)
  arc A1012 (-264.1139, 82.7571) -> (-264.1579, 82.9134) centre (-264.4139, 82.7571) ccw
  arc A1013 (-263.4706, 83.6007) -> (-264.1579, 82.9134) centre (-263.7311, 83.1739) ccw
  arc A1014 (-263.4706, 83.6007) -> (-263.3143, 83.5568) centre (-263.3143, 83.8568) ccw
  line L560 (-263.3143, 83.5568) -> (-262.4139, 83.5568)
  line L561 (-262.4139, 83.5568) -> (-261.5136, 83.5568)
  arc A1015 (-261.5136, 83.5568) -> (-261.3573, 83.6007) centre (-261.5136, 83.8568) ccw
  arc A1016 (-260.67, 82.9134) -> (-261.3573, 83.6007) centre (-261.0968, 83.1739) ccw
  arc A1017 (-260.67, 82.9134) -> (-260.7139, 82.7571) centre (-260.4139, 82.7571) ccw
  line L562 (-260.7139, 82.7571) -> (-260.7139, 82.0568)
  line L563 (-260.7139, 82.0568) -> (-260.7139, 81.3564)
  arc A1018 (-260.7139, 81.3564) -> (-260.67, 81.2001) centre (-260.4139, 81.3564) ccw
  circle A1019 centre (-274.4789, 95.7093) radius 1.5
  circle A1020 centre (-293.5289, 95.7093) radius 1.5
  arc A1021 (-283.2079, 81.2001) -> (-282.5206, 80.5129) centre (-282.7811, 80.9396) ccw
  arc A1022 (-283.2079, 81.2001) -> (-283.1639, 81.3564) centre (-283.4639, 81.3564) ccw
  line L564 (-283.1639, 81.3564) -> (-283.1639, 82.0568)
  line L565 (-283.1639, 82.0568) -> (-283.1639, 82.7571)
  arc A1023 (-283.1639, 82.7571) -> (-283.2079, 82.9134) centre (-283.4639, 82.7571) ccw
  arc A1024 (-282.5206, 83.6007) -> (-283.2079, 82.9134) centre (-282.7811, 83.1739) ccw
  arc A1025 (-282.5206, 83.6007) -> (-282.3643, 83.5568) centre (-282.3643, 83.8568) ccw
  line L566 (-282.3643, 83.5568) -> (-281.4639, 83.5568)
  line L567 (-281.4639, 83.5568) -> (-280.5636, 83.5568)
  arc A1026 (-280.5636, 83.5568) -> (-280.4073, 83.6007) centre (-280.5636, 83.8568) ccw
  arc A1027 (-279.72, 82.9134) -> (-280.4073, 83.6007) centre (-280.1468, 83.1739) ccw
  arc A1028 (-279.72, 82.9134) -> (-279.7639, 82.7571) centre (-279.4639, 82.7571) ccw
  line L568 (-279.7639, 82.7571) -> (-279.7639, 82.0568)
  line L569 (-279.7639, 82.0568) -> (-279.7639, 81.3564)
  arc A1029 (-279.7639, 81.3564) -> (-279.72, 81.2001) centre (-279.4639, 81.3564) ccw
  arc A1030 (-280.4073, 80.5129) -> (-279.72, 81.2001) centre (-280.1468, 80.9396) ccw
  arc A1031 (-280.4073, 80.5129) -> (-280.5636, 80.5568) centre (-280.5635, 80.2571) ccw
  line L570 (-280.5636, 80.5568) -> (-281.4639, 80.5568)
  line L571 (-281.4639, 80.5568) -> (-282.3643, 80.5568)
  arc A1032 (-282.3643, 80.5568) -> (-282.5206, 80.5129) centre (-282.3643, 80.2568) ccw
  arc A1033 (-302.2579, 81.2001) -> (-301.5706, 80.5129) centre (-301.8311, 80.9396) ccw
  arc A1034 (-302.2579, 81.2001) -> (-302.2139, 81.3564) centre (-302.5139, 81.3564) ccw
  line L572 (-302.2139, 81.3564) -> (-302.2139, 82.0568)
  line L573 (-302.2139, 82.0568) -> (-302.2139, 82.7571)
  arc A1035 (-302.2139, 82.7571) -> (-302.2579, 82.9134) centre (-302.5139, 82.7571) ccw
  arc A1036 (-301.5706, 83.6007) -> (-302.2579, 82.9134) centre (-301.8311, 83.1739) ccw
  arc A1037 (-301.5706, 83.6007) -> (-301.4143, 83.5568) centre (-301.4143, 83.8568) ccw
  line L574 (-301.4143, 83.5568) -> (-300.5139, 83.5568)
  line L575 (-300.5139, 83.5568) -> (-299.6136, 83.5568)
  arc A1038 (-299.6136, 83.5568) -> (-299.4573, 83.6007) centre (-299.6136, 83.8568) ccw
  arc A1039 (-298.77, 82.9134) -> (-299.4573, 83.6007) centre (-299.1968, 83.1739) ccw
  arc A1040 (-298.77, 82.9134) -> (-298.8139, 82.7571) centre (-298.5139, 82.7571) ccw
  line L576 (-298.8139, 82.7571) -> (-298.8139, 82.0568)
  line L577 (-298.8139, 82.0568) -> (-298.8139, 81.3564)
  arc A1041 (-298.8139, 81.3564) -> (-298.77, 81.2001) centre (-298.5139, 81.3564) ccw
  arc A1042 (-299.4573, 80.5129) -> (-298.77, 81.2001) centre (-299.1968, 80.9396) ccw
  arc A1043 (-299.4573, 80.5129) -> (-299.6136, 80.5568) centre (-299.6135, 80.2571) ccw
  line L578 (-299.6136, 80.5568) -> (-300.5139, 80.5568)
  line L579 (-300.5139, 80.5568) -> (-301.4143, 80.5568)
  arc A1044 (-301.4143, 80.5568) -> (-301.5706, 80.5129) centre (-301.4143, 80.2568) ccw
  circle A1045 centre (-233.5214, 76.9768) radius 0.875
  circle A1046 centre (-234.7914, 74.4368) radius 1.5
  circle A1047 centre (-238.6014, 76.9768) radius 1.9939
  circle A1048 centre (-243.6814, 76.9768) radius 0.875
  circle A1049 centre (-257.3339, 76.9768) radius 0.875
  circle A1050 centre (-262.4139, 76.9768) radius 1.9939
  circle A1051 centre (-258.6039, 74.4368) radius 1.5
  circle A1052 centre (-241.1414, 71.8968) radius 1.5
  circle A1053 centre (-264.9539, 71.8968) radius 1.5
  circle A1054 centre (-250.5077, 67.4518) radius 1.1
  circle A1055 centre (-267.4939, 76.9768) radius 0.875
  circle A1056 centre (-276.3839, 76.9768) radius 0.875
  circle A1057 centre (-281.4639, 76.9768) radius 1.9939
  circle A1058 centre (-277.6539, 74.4368) radius 1.5
  circle A1059 centre (-286.5439, 76.9768) radius 0.875
  circle A1060 centre (-295.4339, 76.9768) radius 0.875
  circle A1061 centre (-300.5139, 76.9768) radius 1.9939
  circle A1062 centre (-296.7039, 74.4368) radius 1.5
  circle A1063 centre (-284.0039, 71.8968) radius 1.5
  circle A1064 centre (-303.0539, 71.8968) radius 1.5
  arc A1065 (-321.3079, 124.0626) -> (-320.6206, 123.3754) centre (-320.8811, 123.8021) ccw
  arc A1066 (-321.3079, 124.0626) -> (-321.2639, 124.2189) centre (-321.5639, 124.2189) ccw
  line L580 (-321.2639, 124.2189) -> (-321.2639, 124.9193)
  line L581 (-321.2639, 124.9193) -> (-321.2639, 125.6196)
  arc A1067 (-321.2639, 125.6196) -> (-321.3079, 125.7759) centre (-321.5639, 125.6196) ccw
  arc A1068 (-320.6206, 126.4632) -> (-321.3079, 125.7759) centre (-320.8811, 126.0364) ccw
  arc A1069 (-320.6206, 126.4632) -> (-320.4643, 126.4193) centre (-320.4643, 126.7193) ccw
  line L582 (-320.4643, 126.4193) -> (-319.5639, 126.4193)
  line L583 (-319.5639, 126.4193) -> (-318.6636, 126.4193)
  arc A1070 (-318.6636, 126.4193) -> (-318.5073, 126.4632) centre (-318.6636, 126.7193) ccw
  arc A1071 (-317.82, 125.7759) -> (-318.5073, 126.4632) centre (-318.2468, 126.0364) ccw
  arc A1072 (-317.82, 125.7759) -> (-317.8639, 125.6196) centre (-317.5639, 125.6196) ccw
  line L584 (-317.8639, 125.6196) -> (-317.8639, 124.9193)
  line L585 (-317.8639, 124.9193) -> (-317.8639, 124.2189)
  arc A1073 (-317.8639, 124.2189) -> (-317.82, 124.0626) centre (-317.5639, 124.2189) ccw
  arc A1074 (-318.5073, 123.3754) -> (-317.82, 124.0626) centre (-318.2468, 123.8021) ccw
  arc A1075 (-318.5073, 123.3754) -> (-318.6636, 123.4193) centre (-318.6635, 123.1196) ccw
  line L586 (-318.6636, 123.4193) -> (-319.5639, 123.4193)
  line L587 (-319.5639, 123.4193) -> (-320.4643, 123.4193)
  arc A1076 (-320.4643, 123.4193) -> (-320.6206, 123.3754) centre (-320.4643, 123.1193) ccw
  arc A1077 (-340.3579, 124.0626) -> (-339.6706, 123.3754) centre (-339.9311, 123.8021) ccw
  arc A1078 (-340.3579, 124.0626) -> (-340.3139, 124.2189) centre (-340.6139, 124.2189) ccw
  line L588 (-340.3139, 124.2189) -> (-340.3139, 124.9193)
  line L589 (-340.3139, 124.9193) -> (-340.3139, 125.6196)
  arc A1079 (-340.3139, 125.6196) -> (-340.3579, 125.7759) centre (-340.6139, 125.6196) ccw
  arc A1080 (-339.6706, 126.4632) -> (-340.3579, 125.7759) centre (-339.9311, 126.0364) ccw
  arc A1081 (-339.6706, 126.4632) -> (-339.5143, 126.4193) centre (-339.5143, 126.7193) ccw
  line L590 (-339.5143, 126.4193) -> (-338.6139, 126.4193)
  line L591 (-338.6139, 126.4193) -> (-337.7136, 126.4193)
  arc A1082 (-337.7136, 126.4193) -> (-337.5573, 126.4632) centre (-337.7136, 126.7193) ccw
  arc A1083 (-336.87, 125.7759) -> (-337.5573, 126.4632) centre (-337.2968, 126.0364) ccw
  arc A1084 (-336.87, 125.7759) -> (-336.9139, 125.6196) centre (-336.6139, 125.6196) ccw
  line L592 (-336.9139, 125.6196) -> (-336.9139, 124.9193)
  line L593 (-336.9139, 124.9193) -> (-336.9139, 124.2189)
  arc A1085 (-336.9139, 124.2189) -> (-336.87, 124.0626) centre (-336.6139, 124.2189) ccw
  arc A1086 (-337.5573, 123.3754) -> (-336.87, 124.0626) centre (-337.2968, 123.8021) ccw
  arc A1087 (-337.5573, 123.3754) -> (-337.7136, 123.4193) centre (-337.7135, 123.1196) ccw
  line L594 (-337.7136, 123.4193) -> (-338.6139, 123.4193)
  line L595 (-338.6139, 123.4193) -> (-339.5143, 123.4193)
  arc A1088 (-339.5143, 123.4193) -> (-339.6706, 123.3754) centre (-339.5143, 123.1193) ccw
  circle A1089 centre (-305.5939, 119.8393) radius 0.875
  circle A1090 centre (-314.4839, 119.8393) radius 0.875
  circle A1091 centre (-319.5639, 119.8393) radius 1.9939
  circle A1092 centre (-324.6439, 119.8393) radius 0.875
  circle A1093 centre (-315.7539, 117.2993) radius 1.5
  circle A1094 centre (-322.1039, 114.7593) radius 1.5
  circle A1095 centre (-333.5339, 119.8393) radius 0.875
  circle A1096 centre (-334.8039, 117.2993) radius 1.5
  circle A1097 centre (-338.6139, 119.8393) radius 1.9939
  circle A1098 centre (-343.6939, 119.8393) radius 0.875
  circle A1099 centre (-341.1539, 114.7593) radius 1.5
  arc A1100 (-359.4079, 124.0626) -> (-358.7206, 123.3754) centre (-358.9811, 123.8021) ccw
  arc A1101 (-359.4079, 124.0626) -> (-359.3639, 124.2189) centre (-359.6639, 124.2189) ccw
  line L596 (-359.3639, 124.2189) -> (-359.3639, 124.9193)
  line L597 (-359.3639, 124.9193) -> (-359.3639, 125.6196)
  arc A1102 (-359.3639, 125.6196) -> (-359.4079, 125.7759) centre (-359.6639, 125.6196) ccw
  arc A1103 (-358.7206, 126.4632) -> (-359.4079, 125.7759) centre (-358.9811, 126.0364) ccw
  arc A1104 (-358.7206, 126.4632) -> (-358.5643, 126.4193) centre (-358.5643, 126.7193) ccw
  line L598 (-358.5643, 126.4193) -> (-357.6639, 126.4193)
  line L599 (-357.6639, 126.4193) -> (-356.7636, 126.4193)
  arc A1105 (-356.7636, 126.4193) -> (-356.6073, 126.4632) centre (-356.7636, 126.7193) ccw
  arc A1106 (-355.92, 125.7759) -> (-356.6073, 126.4632) centre (-356.3468, 126.0364) ccw
  arc A1107 (-355.92, 125.7759) -> (-355.9639, 125.6196) centre (-355.6639, 125.6196) ccw
  line L600 (-355.9639, 125.6196) -> (-355.9639, 124.9193)
  line L601 (-355.9639, 124.9193) -> (-355.9639, 124.2189)
  arc A1108 (-355.9639, 124.2189) -> (-355.92, 124.0626) centre (-355.6639, 124.2189) ccw
  arc A1109 (-356.6073, 123.3754) -> (-355.92, 124.0626) centre (-356.3468, 123.8021) ccw
  arc A1110 (-356.6073, 123.3754) -> (-356.7636, 123.4193) centre (-356.7635, 123.1196) ccw
  line L602 (-356.7636, 123.4193) -> (-357.6639, 123.4193)
  line L603 (-357.6639, 123.4193) -> (-358.5643, 123.4193)
  arc A1111 (-358.5643, 123.4193) -> (-358.7206, 123.3754) centre (-358.5643, 123.1193) ccw
  arc A1112 (-378.4579, 124.0626) -> (-377.7706, 123.3754) centre (-378.0311, 123.8021) ccw
  arc A1113 (-378.4579, 124.0626) -> (-378.4139, 124.2189) centre (-378.7139, 124.2189) ccw
  line L604 (-378.4139, 124.2189) -> (-378.4139, 124.9193)
  line L605 (-378.4139, 124.9193) -> (-378.4139, 125.6196)
  arc A1114 (-378.4139, 125.6196) -> (-378.4579, 125.7759) centre (-378.7139, 125.6196) ccw
  arc A1115 (-377.7706, 126.4632) -> (-378.4579, 125.7759) centre (-378.0311, 126.0364) ccw
  arc A1116 (-377.7706, 126.4632) -> (-377.6143, 126.4193) centre (-377.6143, 126.7193) ccw
  line L606 (-377.6143, 126.4193) -> (-376.7139, 126.4193)
  line L607 (-376.7139, 126.4193) -> (-375.8136, 126.4193)
  arc A1117 (-375.8136, 126.4193) -> (-375.6573, 126.4632) centre (-375.8136, 126.7193) ccw
  arc A1118 (-374.97, 125.7759) -> (-375.6573, 126.4632) centre (-375.3968, 126.0364) ccw
  arc A1119 (-374.97, 125.7759) -> (-375.0139, 125.6196) centre (-374.7139, 125.6196) ccw
  line L608 (-375.0139, 125.6196) -> (-375.0139, 124.9193)
  line L609 (-375.0139, 124.9193) -> (-375.0139, 124.2189)
  arc A1120 (-375.0139, 124.2189) -> (-374.97, 124.0626) centre (-374.7139, 124.2189) ccw
  arc A1121 (-375.6573, 123.3754) -> (-374.97, 124.0626) centre (-375.3968, 123.8021) ccw
  arc A1122 (-375.6573, 123.3754) -> (-375.8136, 123.4193) centre (-375.8135, 123.1196) ccw
  line L610 (-375.8136, 123.4193) -> (-376.7139, 123.4193)
  line L611 (-376.7139, 123.4193) -> (-377.6143, 123.4193)
  arc A1123 (-377.6143, 123.4193) -> (-377.7706, 123.3754) centre (-377.6143, 123.1193) ccw
  circle A1124 centre (-352.5839, 119.8393) radius 0.875
  circle A1125 centre (-353.8539, 117.2993) radius 1.5
  circle A1126 centre (-357.6639, 119.8393) radius 1.9939
  circle A1127 centre (-362.7439, 119.8393) radius 0.875
  circle A1128 centre (-360.2039, 114.7593) radius 1.5
  circle A1129 centre (-371.6339, 119.8393) radius 0.875
  circle A1130 centre (-372.9039, 117.2993) radius 1.5
  circle A1131 centre (-376.7139, 119.8393) radius 1.9939
  circle A1132 centre (-381.7939, 119.8393) radius 0.875
  circle A1133 centre (-379.2539, 114.7593) radius 1.5
  arc A1134 (-311.7829, 105.0126) -> (-311.0956, 104.3254) centre (-311.3561, 104.7521) ccw
  arc A1135 (-311.7829, 105.0126) -> (-311.7389, 105.1689) centre (-312.0389, 105.1689) ccw
  line L612 (-311.7389, 105.1689) -> (-311.7389, 105.8693)
  line L613 (-311.7389, 105.8693) -> (-311.7389, 106.5696)
  arc A1136 (-311.7389, 106.5696) -> (-311.7829, 106.7259) centre (-312.0389, 106.5696) ccw
  arc A1137 (-311.0956, 107.4132) -> (-311.7829, 106.7259) centre (-311.3561, 106.9864) ccw
  arc A1138 (-311.0956, 107.4132) -> (-310.9393, 107.3693) centre (-310.9393, 107.6693) ccw
  line L614 (-310.9393, 107.3693) -> (-310.0389, 107.3693)
  line L615 (-310.0389, 107.3693) -> (-309.1386, 107.3693)
  arc A1139 (-309.1386, 107.3693) -> (-308.9823, 107.4132) centre (-309.1386, 107.6693) ccw
  arc A1140 (-308.295, 106.7259) -> (-308.9823, 107.4132) centre (-308.7218, 106.9864) ccw
  arc A1141 (-308.295, 106.7259) -> (-308.3389, 106.5696) centre (-308.0389, 106.5696) ccw
  line L616 (-308.3389, 106.5696) -> (-308.3389, 105.8693)
  line L617 (-308.3389, 105.8693) -> (-308.3389, 105.1689)
  arc A1142 (-308.3389, 105.1689) -> (-308.295, 105.0126) centre (-308.0389, 105.1689) ccw
  arc A1143 (-308.9823, 104.3254) -> (-308.295, 105.0126) centre (-308.7218, 104.7521) ccw
  arc A1144 (-308.9823, 104.3254) -> (-309.1386, 104.3693) centre (-309.1385, 104.0696) ccw
  line L618 (-309.1386, 104.3693) -> (-310.0389, 104.3693)
  line L619 (-310.0389, 104.3693) -> (-310.9393, 104.3693)
  arc A1145 (-310.9393, 104.3693) -> (-311.0956, 104.3254) centre (-310.9393, 104.0693) ccw
  arc A1146 (-330.8329, 105.0126) -> (-330.1456, 104.3254) centre (-330.4061, 104.7521) ccw
  arc A1147 (-330.8329, 105.0126) -> (-330.7889, 105.1689) centre (-331.0889, 105.1689) ccw
  line L620 (-330.7889, 105.1689) -> (-330.7889, 105.8693)
  line L621 (-330.7889, 105.8693) -> (-330.7889, 106.5696)
  arc A1148 (-330.7889, 106.5696) -> (-330.8329, 106.7259) centre (-331.0889, 106.5696) ccw
  arc A1149 (-330.1456, 107.4132) -> (-330.8329, 106.7259) centre (-330.4061, 106.9864) ccw
  arc A1150 (-330.1456, 107.4132) -> (-329.9893, 107.3693) centre (-329.9893, 107.6693) ccw
  line L622 (-329.9893, 107.3693) -> (-329.0889, 107.3693)
  line L623 (-329.0889, 107.3693) -> (-328.1886, 107.3693)
  arc A1151 (-328.1886, 107.3693) -> (-328.0323, 107.4132) centre (-328.1886, 107.6693) ccw
  arc A1152 (-327.345, 106.7259) -> (-328.0323, 107.4132) centre (-327.7718, 106.9864) ccw
  arc A1153 (-327.345, 106.7259) -> (-327.3889, 106.5696) centre (-327.0889, 106.5696) ccw
  line L624 (-327.3889, 106.5696) -> (-327.3889, 105.8693)
  line L625 (-327.3889, 105.8693) -> (-327.3889, 105.1689)
  arc A1154 (-327.3889, 105.1689) -> (-327.345, 105.0126) centre (-327.0889, 105.1689) ccw